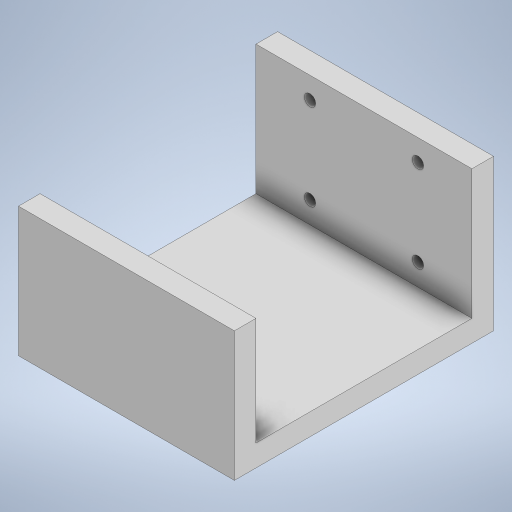
# Autodesk Inventor part: Soporte VNA
Saved by Autodesk Inventor 2024 (Build 280153000, 153)
## iProperties
Created: 2024-06-03
Part Number: Soporte VNA
Material: Generic
Document SubType Name: Modeling
Designer: juanp
Density: 1 g/cm^3
Appearance: Default
Author: juanp
Autodesk Inventor part; units mm, degrees
ref_plane "YZ Plane" through (0, 0, 0) normal (1, 0, 0) x (0, 1, 0)
ref_plane "XZ Plane" through (0, 0, 0) normal (0, 1, 0) x (-1, 0, 0)
ref_plane "XY Plane" through (0, 0, 0) normal (0, 0, 1) x (1, 0, 0)
sketch "Sketch1" plane through (0, 0, 0) normal (0, 0, 1) x (1, 0, 0)
  line L0 (165, -110) -> (-165, -110)
  line L1 (-165, -110) -> (-165, 110)
  line L2 (-165, 110) -> (165, 110)
  line L3 (165, 110) -> (165, -110)
  line L4 (165, -110) -> (-165, 110) construction
  line L5 (-165, -110) -> (165, 110) construction
  point P0 (0, 0)
  dimension "d0" = 330
  dimension "d1" = 220
  constraints: 12 end point, 2 midpoint, 2 parallel, 1 horizontal, 1 perpendicular
  measures "d0" distance of L1.end L2.end
  measures "d1" distance of L0.end L1.end
extrude "Extrusion1" add sketch "Sketch1" along normal blind 100
sketch "Sketch2" plane through (165, -110, 0) normal (1, 0, 0) x (0, 0, -1)
  line L0 (0, 0) -> (0, 220) projected
  line L1 (0, 220) -> (-100, 220) projected
  line L2 (-100, 0) -> (-100, 220) projected
  line L3 (0, 0) -> (-100, 0) projected
  line L4 (-100, 50) -> (-110, 50)
  line L5 (-110, 50) -> (-110, -10)
  line L6 (-110, -10) -> (10, -10)
  line L7 (10, -10) -> (10, 60)
  line L8 (10, 60) -> (0, 60)
  point P0 (0, 110)
  dimension "d4" = 10
  dimension "d5" = 10
  dimension "d6" = 10
  dimension "d7" = 50
  dimension "d8" = 60
  constraints: 10 end point, 4 perpendicular, 2 point on line, 1 horizontal
  measures "d4" distance between parallel lines of L7 L0
  measures "d5" distance between parallel lines of L3 L6
  measures "d6" distance between parallel lines of L5 L2
  measures "d7" distance between parallel lines of L4 L3
  measures "d8" distance between parallel lines of L8 L3
extrude "Extrusion2" add sketch "Sketch2" against normal blind 100 separate body contours L0 L8 L7 L6 L5 L4 L2 L3
sketch "Sketch3" plane through (165, -110, 0) normal (0, 0, 1) x (1, 0, 0)
  line L0 (0, 60) -> (0, 0) projected
  line L1 (0, 60) -> (-100, 60) projected
  line L2 (-100, 0) -> (-100, 60) projected
  line L3 (0, 0) -> (-100, 0) projected
  line L4 (-75, 50) -> (-75, 10) construction
  line L5 (-25, 50) -> (-25, 10) construction
  circle A0 centre (-75, 50) radius 2.65
  circle A1 centre (-75, 10) radius 2.65
  circle A2 centre (-25, 10) radius 2.65
  circle A3 centre (-25, 50) radius 2.65
  line L6 (-75, 30) -> (-25, 30) construction
  line L7 (-50, 30) -> (-50, 60) construction
  line L8 (-50, 0) -> (-50, 30) construction
  point P0 (-165, 110)
  dimension "d11" = 5.3
  dimension "d12" = 40
  dimension "d13" = 50
  constraints: 10 end point, 5 midpoint, 4 centre point, 4 coincident, 3 equal radius, 3 vertical, 2 equal length, 1 horizontal, 1 perpendicular
  measures "d11" diameter of A3
  measures "d12" distance of L5.start L5.end
  measures "d13" distance between parallel lines of L5 L4
extrude "Extrusion3" cut sketch "Sketch3" against normal through all contours A0 | A1 | A2 | A3 bodies 2
body "Solid1"
body "Solid2"
